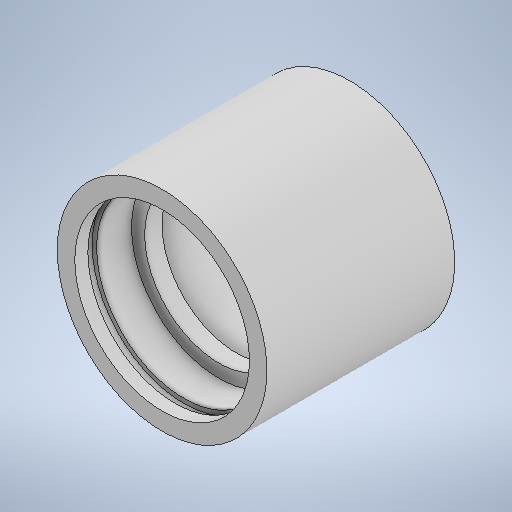
# Autodesk Inventor part: Седло для подшипника
Saved by Autodesk Inventor 2025 (Build 290162010, 162A)
## iProperties
Created: 2024-07-07
Part Number: Седло для подшипника
Material: Generic
Document SubType Name: Modeling
Designer: pokla
Density: 1 g/cm^3
Appearance: Default
Stock Number: Седло для подшипника
Author: pokla
Autodesk Inventor part; units mm, degrees
ref_plane "YZ Plane" through (0, 0, 0) normal (1, 0, 0) x (0, 1, 0)
ref_plane "XZ Plane" through (0, 0, 0) normal (0, 1, 0) x (-1, 0, 0)
ref_plane "XY Plane" through (0, 0, 0) normal (0, 0, 1) x (1, 0, 0)
sketch "Sketch6" plane through (0, 0, 0) normal (0, 0, 1) x (1, 0, 0)
  line L0 (20, 28) -> (24, 28)
  line L1 (24, 28) -> (24, 0)
  line L2 (24, -15) -> (20, -15)
  line L3 (20, -15) -> (20, -12)
  line L4 (17, 2) -> (20, 2)
  line L5 (20, 2) -> (20, -2) construction
  line L6 (20, -2) -> (17, -2)
  line L7 (17, -2) -> (17, 2)
  line L8 (20, -10) -> (21, -10)
  line L9 (21, -10) -> (21, -12)
  line L10 (21, -12) -> (20, -12)
  line L11 (20, -12) -> (20, -10) construction
  line L12 (20, 2) -> (20, 16)
  line L13 (20, -2) -> (20, 2) construction
  line L14 (20, -10) -> (20, -2)
  line L15 (20, -12) -> (20, -10) construction
  line L16 (0, 0) -> (0, 29.8024)
  line L17 (20, 16) -> (21, 16)
  line L18 (21, 16) -> (21, 18)
  line L19 (21, 18) -> (20, 18)
  line L20 (17, 0) -> (24, 0) construction
  line L21 (24, 0) -> (24, -15)
  line L22 (20, 18) -> (20, 28)
  line L23 (20, 16) -> (20, 18) construction
  point P0 (20, 0)
  point P1 (20, -11)
  point P2 (20.5, -10)
  dimension "d15" = 4
  dimension "d16" = 3
  dimension "d17" = 8
  dimension "d18" = 2
  dimension "d19" = 1
  dimension "d21" = 48
  dimension "d22" = 40
  dimension "d24" = 14
  dimension "d25" = 15
  dimension "d26" = 2
  dimension "d27" = 1
  dimension "d28" = 28
  constraints: 48 end point, 19 parallel, 8 perpendicular, 5 horizontal, 4 midpoint, 2 horizontal alignment, 1 vertical, 1 vertical alignment
  measures "d15" distance of L6.end L4.start
  measures "d16" distance of L5.end L6.end
  measures "d17" distance from line of point (20.5, -10) L6
  measures "d18" distance of L8.end L9.end
  measures "d19" distance of L9.end L3.end
  measures "d21" diameter of L1 L16
  measures "d22" diameter of L12 L16
  measures "d24" distance between parallel lines of L17 L4
  measures "d25" distance from line of L1.end L2
  measures "d26" distance of L17.end L18.end
  measures "d27" distance of L12.end L17.end
  measures "d28" distance from line of L1.end L0
revolve "Revolution1" add sketch "Sketch6" angle 360 mid plane about axis through (0, 0, 0) along (0, 1, 0)
equation "\"d26\" = d18"
equation "\"d27\" = d19"
body "Solid2"
